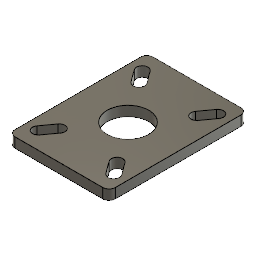
Scoomatic Spacer v2 (Autodesk Fusion 360 design; units mm, degrees)
Autodesk Fusion 360 part; units mm, degrees
sketch "Sketch1" plane through (0, 0, 0) normal (0, 1, 0) x (1, 0, 0)
  line L0 (22.9749, 31.6447) -> (-22.9749, 31.6447) construction
  line L1 (-22.9749, 31.6447) -> (-22.9749, -31.6447) construction
  line L2 (-22.9749, -31.6447) -> (22.9749, -31.6447) construction
  line L3 (22.9749, -31.6447) -> (22.9749, 31.6447) construction
  line L4 (22.9749, 31.6447) -> (-22.9749, -31.6447) construction
  line L5 (-22.9749, 31.6447) -> (22.9749, -31.6447) construction
  line L6 (30.0251, 41.3553) -> (-30.0251, 41.3553) construction
  line L7 (-30.0251, 41.3553) -> (-30.0251, -41.3553) construction
  line L8 (-30.0251, -41.3553) -> (30.0251, -41.3553) construction
  line L9 (30.0251, -41.3553) -> (30.0251, 41.3553) construction
  line L10 (30.0251, 41.3553) -> (-30.0251, -41.3553) construction
  line L11 (-30.0251, 41.3553) -> (30.0251, -41.3553) construction
  line L12 (26.6164, 29.0009) -> (33.6665, 38.7115)
  arc A0 (33.6665, 38.7115) -> (26.3836, 43.9991) centre (30.0251, 41.3553) ccw
  line L13 (26.3836, 43.9991) -> (19.3335, 34.2885)
  arc A1 (19.3335, 34.2885) -> (26.6164, 29.0009) centre (22.9749, 31.6447) ccw
  line L14 (22.9749, 31.6447) -> (30.0251, 41.3553) construction
  line L15 (0, 0) -> (0, 52.4802) construction
  line L16 (0, 0) -> (-40, 0) construction
  arc A2 (-26.3836, 43.9991) -> (-33.6665, 38.7115) centre (-30.0251, 41.3553) ccw
  line L17 (-26.6164, 29.0009) -> (-33.6665, 38.7115)
  arc A3 (-26.6164, 29.0009) -> (-19.3335, 34.2885) centre (-22.9749, 31.6447) ccw
  line L18 (-26.3836, 43.9991) -> (-19.3335, 34.2885)
  arc A4 (-33.6665, -38.7115) -> (-26.3836, -43.9991) centre (-30.0251, -41.3553) ccw
  line L19 (-26.3836, -43.9991) -> (-19.3335, -34.2885)
  line L20 (-26.6164, -29.0009) -> (-33.6665, -38.7115)
  arc A5 (-19.3335, -34.2885) -> (-26.6164, -29.0009) centre (-22.9749, -31.6447) ccw
  line L21 (26.3836, -43.9991) -> (19.3335, -34.2885)
  arc A6 (26.3836, -43.9991) -> (33.6665, -38.7115) centre (30.0251, -41.3553) ccw
  line L22 (26.6164, -29.0009) -> (33.6665, -38.7115)
  arc A7 (26.6164, -29.0009) -> (19.3335, -34.2885) centre (22.9749, -31.6447) ccw
  line L23 (39.9315, 55) -> (-39.9315, 55)
  line L24 (-39.9315, 55) -> (-39.9315, -55)
  line L25 (-39.9315, -55) -> (39.9315, -55)
  line L26 (39.9315, -55) -> (39.9315, 55)
  line L27 (39.9315, 55) -> (-39.9315, -55) construction
  line L28 (-39.9315, 55) -> (39.9315, -55) construction
  circle A8 centre (0, 0) radius 16.5
  line L29 (26.5, 36.5) -> (24.038, 38.2875) construction
  point P0 (26.5, 36.5)
  point P1 (-26.5, 36.5)
  point P2 (26.5, -36.5)
  point P3 (-26.5, -36.5)
  dimension "d1" = 4.5
  dimension "d2" = 12
  dimension "d5" = 110
  dimension "d9" = 33
  dimension "d11" = 73
  dimension "d13" = 53
  constraint perpendicular L0 L1
  constraint parallel L0 L2
  constraint parallel L1 L3
  constraint horizontal L0
  constraint coincident L4 L15.start
  constraint coincident L5 L15.start
  constraint coincident L15.start L16.start
  constraint perpendicular L6 L7
  constraint parallel L6 L8
  constraint parallel L7 L9
  constraint horizontal L6
  constraint coincident L10 L15.start
  constraint coincident L11 L15.start
  constraint collinear L4 L10
  constraint tangent L12 A0
  constraint tangent A0 L13
  constraint parallel L12 L13
  constraint tangent L13 A1
  constraint tangent L12 A1
  constraint coincident L6.start L9.end
  constraint parallel L10 L14
  constraint coincident L0.start L3.end
  constraint vertical L15
  constraint perpendicular L15 L16
  constraint symmetric L12.start L15 L17.start
  constraint symmetric L12.end L15 A2.end
  constraint symmetric A0.end L15 A2.start
  constraint symmetric L13.end L15 A3.end
  constraint symmetric A0 L15 A2
  constraint symmetric A1 L15 A3
  constraint symmetric L12.start L16 L22.start
  constraint symmetric L12.end L16 A6.end
  constraint symmetric A0.end L16 L21.start
  constraint symmetric L13.end L16 L21.end
  constraint symmetric A0 L16 A6
  constraint symmetric A1 L16 A7
  constraint symmetric L16 A2.end A4.start
  constraint symmetric L16 A2.start A4.end
  constraint symmetric L16 A2 A4
  constraint symmetric L16 L17.start L20.start
  constraint symmetric L16 A3.end L19.end
  constraint symmetric L16 A3 A5
  constraint perpendicular L23 L24
  constraint parallel L23 L25
  constraint parallel L24 L26
  constraint horizontal L23
  constraint coincident L27 L15.start
  constraint coincident L28 L15.start
  constraint collinear L4 L27
  constraint coincident L14 P0
  constraint symmetric L15 P0 P1
  constraint symmetric L16 P0 P2
  constraint symmetric L16 P1 P3
  constraint coincident P0 L29.start
  constraint perpendicular L27 L29
  constraint symmetric L0.start L6.start L29
  measures "d1" radius of A0
  measures "d2" distance of L0.start L6.start
  measures "d5" distance of L23 L25
  measures "d9" diameter of A8
  measures "d11" distance of P0 P2
  measures "d13" distance of P2 P3
extrude "Extrude1" add sketch "Sketch1" along normal blind 8
fillet "Fillet1" radius 5 4 edges at (39.9315, 4, -55) (-39.9315, 4, 55) (39.9315, 4, 55) (-39.9315, 4, -55)
equation "d1 = ( 9 / 2 ) * 1 mm"
